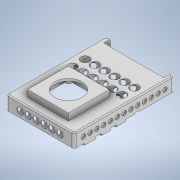
# Autodesk Inventor part: Pi 4 Case  - Upper Panel
Saved by Autodesk Inventor 2020 (Build 240168000, 168)
## iProperties
Created: 2021-01-01
Part Number: Pi 4 Case  - Upper Panel
Material: Generic
Document SubType Name: Modeling
Designer: frost
Density: 1 g/cm^3
Appearance: Default
Author: frost
Autodesk Inventor part; units mm, degrees
ref_plane "YZ Plane" through (0, 0, 0) normal (1, 0, 0) x (0, 1, 0)
ref_plane "XZ Plane" through (0, 0, 0) normal (0, 1, 0) x (-1, 0, 0)
sketch "Sketch1" plane through (0, 0, 0) normal (0, 1, 0) x (-1, 0, 0)
  line L0 (28, 44) -> (-28, 44)
  line L1 (-30, 42) -> (-30, -42)
  line L2 (-28, -44) -> (28, -44)
  line L3 (30, -42) -> (30, 42)
  line L4 (30, 44) -> (-30, -44) construction
  line L5 (-30, 44) -> (30, -44) construction
  line L6 (25, 42.5) -> (-25, 42.5)
  line L7 (-28, 39.5) -> (-28, -39.5)
  line L8 (-25, -42.5) -> (25, -42.5)
  line L9 (28, -39.5) -> (28, 39.5)
  line L10 (28, 42.5) -> (-28, -42.5) construction
  line L11 (-28, 42.5) -> (28, -42.5) construction
  arc A0 (25, -42.5) -> (28, -39.5) centre (25, -39.5) ccw
  arc A1 (-28, -39.5) -> (-25, -42.5) centre (-25, -39.5) ccw
  arc A2 (-25, 42.5) -> (-28, 39.5) centre (-25, 39.5) ccw
  arc A3 (28, 39.5) -> (25, 42.5) centre (25, 39.5) ccw
  arc A4 (-30, -42) -> (-28, -44) centre (-28, -42) ccw
  arc A5 (-28, 44) -> (-30, 42) centre (-28, 42) ccw
  arc A6 (28, -44) -> (30, -42) centre (28, -42) ccw
  arc A7 (30, 42) -> (28, 44) centre (28, 42) ccw
  point P0 (0, 0)
  dimension "d2" = 60
  dimension "d3" = 88
  dimension "d4" = 56
  dimension "d5" = 85
  dimension "d6" = 3
  dimension "d7" = 2
  constraints: 24 end point, 16 point on circle, 16 point on line, 16 tangent, 8 centre point, 6 equal radius, 4 midpoint, 4 parallel, 2 horizontal, 2 perpendicular
  measures "d2" distance of L4.end L5.end
  measures "d3" distance of L5.start L4.end
  measures "d4" distance of L11.end L10.end
  measures "d5" distance of L10.end L11.start
  measures "d6" radius of A0
  measures "d7" radius of A4
extrude "Extrusion1" add sketch "Sketch1" along normal blind 4 contours A7 L3 A6 L2 A4 L1 A5 L0 | A3 L9 A0 L8 A1 L7 A2 L6
extrude "Extrusion2" add sketch "Sketch1" against normal blind 8
sketch "Sketch2" plane through (28, 4, -44) normal (0, 0, -1) x (-1, 0, 0)
  line L0 (53, -12) -> (3, -12) projected
  line L1 (2, -1) -> (54, -1)
  line L2 (54, -1) -> (54, -12)
  line L3 (54, -12) -> (2, -12)
  line L4 (2, -12) -> (2, -1)
  line L5 (-2, -12) -> (-2, 0) projected
  line L6 (58, -12) -> (58, 0) projected
  point P0 (28, -4)
  point P1 (3, -12)
  dimension "d12" = 4
  dimension "d13" = 4
  dimension "d14" = 11
  constraints: 8 end point, 2 parallel, 1 horizontal, 1 perpendicular, 1 point on line
  measures "d12" distance between parallel lines of L5 L4
  measures "d13" distance between parallel lines of L6 L2
  measures "d14" distance of L1.end L2.end
extrude "Extrusion3" cut sketch "Sketch2" against normal blind 19
sketch "Sketch3" plane through (28, 4, -44) normal (0, 0, -1) x (-1, 0, 0)
  line L0 (2, -1) -> (54, -1) projected
  line L1 (54, -1) -> (38, -1)
  line L2 (38, -1) -> (38, -3.5)
  line L3 (38, -3.5) -> (54, -3.5)
  line L4 (54, -3.5) -> (54, -1)
  line L5 (0, 0) -> (56, 0) projected
  line L6 (2, -1) -> (54, -1)
  line L7 (54, -1) -> (54, 0)
  line L8 (54, 0) -> (2, 0)
  line L9 (2, 0) -> (2, -1)
  point P0 (28, -4)
  point P1 (38, -1)
  dimension "d67" = 6
  dimension "d17" = 16
  dimension "d18" = 2.5
  constraints: 16 end point, 4 parallel, 2 horizontal, 2 perpendicular, 1 point on line
  measures "d17" distance of L3.end L2.end
  measures "d18" distance of L2.end L1.end
extrude "Extrusion4" add sketch "Sketch3" against normal blind 21 contours L0 L4 L3 L2
extrude "Extrusion5" cut sketch "Sketch3" against normal blind 5
sketch "Sketch4" plane through (30, 4, 42) normal (1, 0, 0) x (0, 0, -1)
  line L0 (86, -12) -> (86, 0) projected
  line L1 (84, -12) -> (0, -12) projected
  circle A0 centre (53.5, -14.5) radius 3.5
  point P0 (42, -4)
  point P1 (51.05051, -12)
  point P2 (55.94949, -12)
  dimension "d27" = 2.5
  dimension "d28" = 32.5
  dimension "d29" = 7
  constraints: 1 centre point
  measures "d27" distance from line of L1 A0.centre
  measures "d28" distance from line of L0 A0.centre
  measures "d29" diameter of A0
extrude "Extrusion6" cut sketch "Sketch4" against normal blind 10 contours L1 A0 picked at (52.886513, -11.84099)
sketch "Sketch5" plane through (30, 4, 42) normal (1, 0, 0) x (0, 0, -1)
  line L0 (-4.909383, -13.7) -> (89.753099, -13.7)
  line L1 (84, -12) -> (55.94949, -12)
  point P0 (42, -4)
  dimension "d32" = 1.7
  constraints: 2 end point, 1 horizontal
  measures "d32" distance between parallel lines of L1 L0
sketch "Sketch6" plane through (30, 4, 42) normal (1, 0, 0) x (0, 0, -1)
  line L0 (43, -10.06382) -> (43, -13.7)
  arc A0 (55.94949, -12) -> (51.05051, -12) centre (53.5, -14.5) ccw
  line L1 (35, -10.06382) -> (35, -13.7)
  line L2 (30, -13.7) -> (30, -10.06382)
  line L3 (22, -10.06382) -> (22, -13.7)
  line L4 (17, -10.06382) -> (17, -13.7)
  line L5 (7, -10.06382) -> (7, -13.7)
  line L6 (6.470177, -10.06382) -> (43, -10.06382)
  line L7 (-3.727507, -13.7) -> (104.881709, -13.7)
  line L8 (84, -12) -> (55.94949, -12)
  point P0 (42, -4)
  dimension "d33" = 10.5
  dimension "d34" = 8
  dimension "d35" = 5
  dimension "d36" = 8
  dimension "d37" = 5
  dimension "d38" = 10
  dimension "d39" = 1.7
  constraints: 16 end point, 11 point on line, 6 vertical, 2 horizontal
  measures "d33" distance from line of L0 A0.centre
  measures "d34" distance between parallel lines of L0 L1
  measures "d35" distance between parallel lines of L1 L2
  measures "d36" distance between parallel lines of L3 L2
  measures "d37" distance between parallel lines of L4 L3
  measures "d38" distance between parallel lines of L4 L5
  measures "d39" distance between parallel lines of L8 L7
extrude "Extrusion7" add sketch "Sketch6" against normal blind 2 contours L0 L7 L1 L6 | L2 L7 L3 L6 | L4 L7 L5 L6
fillet "Fillet1" radius 1 11 edges at (29.4142, 4, -43.4142) (27, 4, -44) (29.4142, 4, 43.4142) (0, 4, 44) (-29.4142, 4, 43.4142) (-30, 4, 0) (-29.4142, 4, -43.4142) (-27, 4, -44) (30, 4, 0) (0, 4, -39) (26, 4, -41.5)
sketch "Sketch8" plane through (0, 0, 0) normal (0, -1, 0) x (1, 0, 0)
  line L0 (28, 44) -> (-28, 44)
  line L1 (0, 44) -> (0, 19)
  line L2 (0, 19) -> (12.020815, 31.020815)
  line L3 (0, 19) -> (16.563989, 19)
  line L4 (0, 19) -> (-12.020815, 31.020815)
  line L5 (0, 19) -> (12.020815, 6.979185)
  line L6 (0, 19) -> (-12.020815, 6.979185)
  circle A0 centre (12.020815, 31.020815) radius 1.25
  circle A1 centre (-12.020815, 31.020815) radius 1.25
  circle A2 centre (12.020815, 6.979185) radius 1.25
  circle A3 centre (-12.020815, 6.979185) radius 1.25
  line L7 (17, 36) -> (-17, 36)
  line L8 (-17, 36) -> (-17, 2)
  line L9 (-17, 2) -> (17, 2)
  line L10 (17, 2) -> (17, 36)
  line L11 (17, 36) -> (-17, 2) construction
  line L12 (-17, 36) -> (17, 2) construction
  line L13 (18, 37) -> (-18, 37)
  line L14 (-18, 37) -> (-18, 1)
  line L15 (-18, 1) -> (18, 1)
  line L16 (18, 1) -> (18, 37)
  line L17 (18, 37) -> (-18, 1) construction
  line L18 (-18, 37) -> (18, 1) construction
  circle A4 centre (-12.020815, 6.979185) radius 2.5
  circle A5 centre (-12.020815, 31.020815) radius 2.5
  circle A6 centre (12.020815, 31.020815) radius 2.5
  circle A7 centre (12.020815, 6.979185) radius 2.5
  point P0 (0, 0)
  dimension "d43" = 25
  dimension "d44" = 17
  dimension "d45" = 45
  dimension "d46" = 2.5
  dimension "d47" = 2.5
  dimension "d48" = 34
  dimension "d49" = 34
  dimension "d50" = 36
  dimension "d51" = 36
  dimension "d56" = 5
  dimension "d57" = 5
  dimension "d58" = 5
  dimension "d59" = 5
  constraints: 36 end point, 8 centre point, 5 coincident, 5 midpoint, 5 symmetric about line, 4 parallel, 3 horizontal, 2 perpendicular, 1 point on line, 1 vertical, 2 other
  measures "d43" distance of L1.start L1.end
  measures "d44" distance of L1.end L2.end
  measures "d45" angle of L1 L2
  measures "d46" diameter of A0
  measures "d47" diameter of A1
  measures "d48" distance of L9.end L8.end
  measures "d49" distance of L8.end L7.end
  measures "d50" distance of L15.end L14.end
  measures "d51" distance of L15.end L13.start
  measures "d56" diameter of A4
  measures "d57" diameter of A5
  measures "d58" diameter of A6
  measures "d59" diameter of A7
extrude "Extrusion8" add sketch "Sketch8" against normal blind 10 contours A0 | A1 | A2 | A3 | L10 L9 L8 L7 | L16 L15 L14 L13 | A4 | A5 | A6 | A7
extrude "Extrusion9" cut sketch "Sketch8" against normal blind 8 contours A0 | A1 | A2 | A3 | L10 L9 L8 L7 | A4 | A5 | A6 | A7
extrude "Extrusion10" add sketch "Sketch8" against normal blind 8 contours A4 | A5 | A6 | A7
extrude "Extrusion11" cut sketch "Sketch8" against normal blind 4 contours A4 | A5 | A6 | A7
sketch "Sketch9" plane through (0, 10, 0) normal (0, 1, 0) x (1, 0, 0)
  circle A0 centre (12.020815, -31.020815) radius 1.25
  circle A1 centre (-12.020815, -6.979185) radius 1.25
  line L0 (12.020815, -31.020815) -> (-12.020815, -6.979185)
  circle A2 centre (0, -19) radius 12
  point P0 (0, 0)
  dimension "d64" = 24
  constraints: 2 end point, 1 centre point, 1 midpoint
  measures "d64" diameter of A2
extrude "Extrusion12" cut sketch "Sketch9" against normal blind 4 contours A2 L0 | L0 A2
sketch "Sketch10" plane through (-30, -8, -42) normal (-1, 0, 0) x (0, 0, 1)
  line L0 (84, 11) -> (0, 11)
  line L1 (0, 11) -> (0, 0)
  line L2 (2.5, 0) -> (-0.328427, 0)
  line L3 (0, 0) -> (0, 11)
  line L4 (0, 5.5) -> (132, 5.5)
  circle A0 centre (6, 5.5) radius 2
  circle A1 centre (12, 5.5) radius 2
  circle A2 centre (18, 5.5) radius 2
  circle A3 centre (24, 5.5) radius 2
  circle A4 centre (30, 5.5) radius 2
  circle A5 centre (36, 5.5) radius 2
  circle A6 centre (42, 5.5) radius 2
  circle A7 centre (48, 5.5) radius 2
  circle A8 centre (54, 5.5) radius 2
  circle A9 centre (60, 5.5) radius 2
  circle A10 centre (66, 5.5) radius 2
  circle A11 centre (72, 5.5) radius 2
  circle A12 centre (78, 5.5) radius 2
  line L5 (84, 0) -> (84, 11)
  circle A13 centre (9, 5.5) radius 2
  circle A14 centre (15, 5.5) radius 2
  circle A15 centre (21, 5.5) radius 2
  circle A16 centre (27, 5.5) radius 2
  circle A17 centre (33, 5.5) radius 2
  circle A18 centre (39, 5.5) radius 2
  circle A19 centre (45, 5.5) radius 2
  circle A20 centre (51, 5.5) radius 2
  circle A21 centre (57, 5.5) radius 2
  circle A22 centre (63, 5.5) radius 2
  circle A23 centre (69, 5.5) radius 2
  circle A24 centre (75, 5.5) radius 2
  circle A25 centre (81, 5.5) radius 2
  circle A26 centre (3, 5.5) radius 2
  point P0 (42, 8)
  dimension "d67" = 6
  dimension "d68" = 6
  dimension "d69" = 6
  dimension "d70" = 6
  dimension "d71" = 6
  dimension "d72" = 6
  dimension "d73" = 6
  dimension "d74" = 6
  dimension "d75" = 6
  dimension "d76" = 6
  dimension "d77" = 6
  dimension "d78" = 6
  dimension "d79" = 6
  dimension "d80" = 4
  dimension "d81" = 3
  dimension "d82" = 3
  dimension "d83" = 3
  dimension "d84" = 3
  dimension "d85" = 3
  dimension "d86" = 3
  dimension "d87" = 3
  dimension "d88" = 3
  dimension "d89" = 3
  dimension "d90" = 3
  dimension "d91" = 3
  dimension "d92" = 3
  dimension "d93" = 3
  dimension "d94" = 3
  constraints: 27 centre point, 26 equal radius, 2 end point, 1 midpoint, 1 point on line, 1 vertical, 30 other
  measures "d67" distance from line of L1 A0.centre
  measures "d68" distance of A0.centre A1.centre
  measures "d69" distance from line of L5 A12.centre
  measures "d70" distance of A12.centre A11.centre
  measures "d71" distance of A11.centre A10.centre
  measures "d72" distance of A10.centre A9.centre
  measures "d73" distance of A9.centre A8.centre
  measures "d74" distance of A8.centre A7.centre
  measures "d75" distance of A7.centre A6.centre
  measures "d76" distance of A6.centre A5.centre
  measures "d77" distance of A5.centre A4.centre
  measures "d78" distance of A4.centre A3.centre
  measures "d79" distance of A3.centre A2.centre
  measures "d80" diameter of A0
  measures "d81" distance of A0.centre A26.centre
  measures "d82" distance of A1.centre A13.centre
  measures "d83" distance of A2.centre A14.centre
  measures "d84" distance of A3.centre A15.centre
  measures "d85" distance of A4.centre A16.centre
  measures "d86" distance of A5.centre A17.centre
  measures "d87" distance of A6.centre A18.centre
  measures "d88" distance of A7.centre A19.centre
  measures "d89" distance of A8.centre A20.centre
  measures "d90" distance of A9.centre A21.centre
  measures "d91" distance of A10.centre A22.centre
  measures "d92" distance of A11.centre A23.centre
  measures "d93" distance of A12.centre A24.centre
  measures "d94" distance of A12.centre A25.centre
extrude "Extrusion13" cut sketch "Sketch10" against normal blind 3 contours A25 A12 L4 | L4 A12 A25 | A26 A0 L4 | L4 A0 A26 | A12 A25 L4 | L4 A25 A12 | A0 A26 L4 | L4 A26 A0 | A24 L4 A12 | A12 L4 A11 A24 | A24 A11 L4 A12 | A12 L4 A24 | A13 A1 L4 A0 | A0 L4 A13 | A13 L4 A0 | A0 L4 A1 A13 | A11 L4 A24 | A24 L4 A11 | A13 L4 A1 | A1 L4 A13 | A23 L4 A11 | A11 L4 A10 A23 | A23 A10 L4 A11 | A11 L4 A23 | A14 A2 L4 A1 | A1 L4 A14 | A14 L4 A1 | A1 L4 A2 A14 | A10 L4 A23 | A23 L4 A10 | A14 L4 A2 | A2 L4 A14 | A22 L4 A10 | A10 L4 A9 A22 | A22 A9 L4 A10 | A10 L4 A22 | A15 A3 L4 A2 | A2 L4 A15 | A15 L4 A2 | A2 L4 A3 A15 | A9 L4 A22 | A22 L4 A9 | A15 L4 A3 | A3 L4 A15 | A21 L4 A9 | A9 L4 A8 A21 | A21 A8 L4 A9 | A9 L4 A21 | A16 A4 L4 A3 | A3 L4 A16 | A16 L4 A3 | A3 L4 A4 A16 | A8 L4 A21 | A21 L4 A8 | A16 L4 A4 | A4 L4 A16 | A20 L4 A8 | A8 L4 A7 A20 | A20 A7 L4 A8 | A8 L4 A20 | A17 A5 L4 A4 | A4 L4 A17 | A17 L4 A4 | A4 L4 A5 A17 | A7 L4 A20 | A20 L4 A7 | A17 L4 A5 | A5 L4 A17 | A19 L4 A7 | A7 L4 A6 A19 | A19 A6 L4 A7 | A7 L4 A19 | A18 A6 L4 A5 | A5 L4 A18 | A18 L4 A5 | A5 L4 A6 A18 | A6 L4 A19 | A19 L4 A6 | A18 L4 A6 | A6 L4 A18
extrude "Extrusion14" add sketch "Sketch10" against normal blind 1 contours A25 A12 L4 | L4 A12 A25 | A26 A0 L4 | L4 A0 A26 | A12 A25 L4 | L4 A25 A12 | A0 A26 L4 | L4 A26 A0 | A24 L4 A12 | A12 L4 A11 A24 | A24 A11 L4 A12 | A12 L4 A24 | A13 A1 L4 A0 | A0 L4 A13 | A13 L4 A0 | A0 L4 A1 A13 | A11 L4 A24 | A24 L4 A11 | A13 L4 A1 | A1 L4 A13 | A23 L4 A11 | A11 L4 A10 A23 | A23 A10 L4 A11 | A11 L4 A23 | A14 A2 L4 A1 | A1 L4 A14 | A14 L4 A1 | A1 L4 A2 A14 | A10 L4 A23 | A23 L4 A10 | A14 L4 A2 | A2 L4 A14 | A22 L4 A10 | A10 L4 A9 A22 | A22 A9 L4 A10 | A10 L4 A22 | A15 A3 L4 A2 | A2 L4 A15 | A15 L4 A2 | A2 L4 A3 A15 | A9 L4 A22 | A22 L4 A9 | A15 L4 A3 | A3 L4 A15 | A21 L4 A9 | A9 L4 A8 A21 | A21 A8 L4 A9 | A9 L4 A21 | A16 A4 L4 A3 | A3 L4 A16 | A16 L4 A3 | A3 L4 A4 A16 | A8 L4 A21 | A21 L4 A8 | A16 L4 A4 | A4 L4 A16 | A20 L4 A8 | A8 L4 A7 A20 | A20 A7 L4 A8 | A8 L4 A20 | A17 A5 L4 A4 | A4 L4 A17 | A17 L4 A4 | A4 L4 A5 A17 | A7 L4 A20 | A20 L4 A7 | A17 L4 A5 | A5 L4 A17 | A19 L4 A7 | A7 L4 A6 A19 | A19 A6 L4 A7 | A7 L4 A19 | A18 A6 L4 A5 | A5 L4 A18 | A18 L4 A5 | A5 L4 A6 A18 | A6 L4 A19 | A19 L4 A6 | A18 L4 A6 | A6 L4 A18
extrude "Extrusion15" cut sketch "Sketch10" against normal blind 1 contours A12 A25 L4 | L4 A25 A12 | A25 L4 A24 A12 | A12 A24 L4 A25 | A0 A26 L4 | L4 A26 A0 | A0 A13 L4 A26 | A26 L4 A13 A0 | A24 L4 A12 | A12 L4 A24 | A0 L4 A13 | A13 L4 A0 | A24 L4 A23 A11 | A11 L4 A24 | A24 L4 A11 | A11 A23 L4 A24 | A13 L4 A1 | A1 A14 L4 A13 | A13 L4 A14 A1 | A1 L4 A13 | A23 L4 A11 | A11 L4 A23 | A1 L4 A14 | A14 L4 A1 | A23 L4 A22 A10 | A10 L4 A23 | A23 L4 A10 | A10 A22 L4 A23 | A14 L4 A2 | A2 A15 L4 A14 | A14 L4 A15 A2 | A2 L4 A14 | A22 L4 A10 | A10 L4 A22 | A2 L4 A15 | A15 L4 A2 | A22 L4 A21 A9 | A9 L4 A22 | A22 L4 A9 | A9 A21 L4 A22 | A15 L4 A3 | A3 A16 L4 A15 | A15 L4 A16 A3 | A3 L4 A15 | A21 L4 A9 | A9 L4 A21 | A3 L4 A16 | A16 L4 A3 | A21 L4 A20 A8 | A8 L4 A21 | A21 L4 A8 | A8 A20 L4 A21 | A16 L4 A4 | A4 A17 L4 A16 | A16 L4 A17 A4 | A4 L4 A16 | A20 L4 A8 | A8 L4 A20 | A4 L4 A17 | A17 L4 A4 | A20 L4 A19 A7 | A7 L4 A20 | A20 L4 A7 | A7 A19 L4 A20 | A17 L4 A5 | A5 A18 L4 A17 | A17 L4 A18 A5 | A5 L4 A17 | A19 L4 A7 | A7 L4 A19 | A5 L4 A18 | A18 L4 A5 | A19 L4 A18 A6 | A6 L4 A19 | A19 L4 A6 | A6 A18 L4 A19 | A18 L4 A6 | A6 L4 A18 picked at (79.352586, 5.340941) picked at (79.352586, 5.659059) picked at (4.352586, 5.659059) picked at (4.352586, 5.340941)
ref_plane "Work Plane1" through (0, -8, -42) normal (-1, 0, 0) x (0, 0, 1)
mirror "Mirror1" about plane through (0, -8, -42) normal (-1, 0, 0) of "Extrusion15", "Extrusion14", "Extrusion13"
sketch "Sketch11" plane through (-28, -8, 44) normal (0, 0, 1) x (1, 0, 0)
  line L0 (0, 11) -> (-2, 11)
  line L1 (0, 0) -> (0, 11)
  line L2 (0, 11) -> (0, 0)
  line L3 (0, 7.5) -> (0, 3.5)
  line L4 (0, 5.5) -> (67.775068, 5.5)
  circle A0 centre (7, 5.5) radius 3
  circle A1 centre (14, 5.5) radius 3
  circle A2 centre (21, 5.5) radius 3
  circle A3 centre (28, 5.5) radius 3
  circle A4 centre (35, 5.5) radius 3
  circle A5 centre (42, 5.5) radius 3
  circle A6 centre (49, 5.5) radius 3
  line L5 (56, 11) -> (56, 0)
  circle A7 centre (45.5, 5.5) radius 3
  circle A8 centre (38.5, 5.5) radius 3
  circle A9 centre (31.5, 5.5) radius 3
  circle A10 centre (24.5, 5.5) radius 3
  circle A11 centre (10.5, 5.5) radius 3
  circle A12 centre (17.5, 5.5) radius 3
  point P0 (28, 8)
  dimension "d101" = 7
  dimension "d102" = 7
  dimension "d103" = 7
  dimension "d104" = 7
  dimension "d105" = 7
  dimension "d106" = 7
  dimension "d107" = 7
  dimension "d108" = 6
  dimension "d109" = 3.5
  dimension "d110" = 3.5
  dimension "d111" = 3.5
  dimension "d112" = 3.5
  dimension "d113" = 3.5
  dimension "d114" = 3.5
  constraints: 13 centre point, 12 equal radius, 2 end point, 1 collinear, 1 midpoint, 16 other
  measures "d101" distance from line of L1 A0.centre
  measures "d102" distance of A1.centre A0.centre
  measures "d103" distance of A1.centre A2.centre
  measures "d104" distance from line of L5 A6.centre
  measures "d105" distance of A6.centre A5.centre
  measures "d106" distance of A5.centre A4.centre
  measures "d107" distance of A4.centre A3.centre
  measures "d108" diameter of A0
  measures "d109" distance of A1.centre A11.centre
  measures "d110" distance of A2.centre A12.centre
  measures "d111" distance of A3.centre A10.centre
  measures "d112" distance of A4.centre A9.centre
  measures "d113" distance of A5.centre A8.centre
  measures "d114" distance of A6.centre A7.centre
extrude "Extrusion16" cut sketch "Sketch11" against normal blind 1.5 contours A7 A6 L4 | A7 A6 L4 | L4 A6 A7 | L4 A6 A7 | A5 A7 L4 | L4 A7 A5 | A7 L4 A8 A5 | A5 A8 L4 A7 | A8 L4 A5 | A5 L4 A8 | A8 L4 A9 A4 | A4 L4 A8 | A8 L4 A4 | A4 A9 L4 A8 | A9 L4 A4 | A4 L4 A9 | A9 L4 A10 A3 | A3 L4 A9 | A9 L4 A3 | A3 A10 L4 A9 | A10 L4 A3 | A3 L4 A10 | A10 L4 A12 A2 | A2 L4 A10 | A10 L4 A2 | A2 A12 L4 A10 | A12 L4 A2 | A2 L4 A12 | A12 L4 A11 A1 | A1 L4 A12 | A12 L4 A1 | A1 A11 L4 A12 | A11 L4 A1 | A1 L4 A11 | A11 L4 A0 | A0 L4 A11 | A11 L4 A0 | A0 L4 A11
extrude "Extrusion17" add sketch "Sketch11" against normal blind 0.75 contours A7 A6 L4 | A7 A6 L4 | L4 A6 A7 | L4 A6 A7 | A5 A7 L4 | L4 A7 A5 | A7 L4 A8 A5 | A5 A8 L4 A7 | A8 L4 A5 | A5 L4 A8 | A8 L4 A9 A4 | A4 L4 A8 | A8 L4 A4 | A4 A9 L4 A8 | A9 L4 A4 | A4 L4 A9 | A9 L4 A10 A3 | A3 L4 A9 | A9 L4 A3 | A3 A10 L4 A9 | A10 L4 A3 | A3 L4 A10 | A10 L4 A12 A2 | A2 L4 A10 | A10 L4 A2 | A2 A12 L4 A10 | A12 L4 A2 | A2 L4 A12 | A12 L4 A11 A1 | A1 L4 A12 | A12 L4 A1 | A1 A11 L4 A12 | A11 L4 A1 | A1 L4 A11 | A11 L4 A0 | A0 L4 A11 | A11 L4 A0 | A0 L4 A11
extrude "Extrusion18" cut sketch "Sketch11" against normal blind 0.75 contours A7 A6 L4 | L4 A6 A7 | A6 A7 A5 L4 | L4 A5 A7 A6 | A5 A7 L4 | L4 A7 A5 | A8 L4 A5 | A5 L4 A4 A8 | A8 A4 L4 A5 | A5 L4 A8 | A4 L4 A8 | A8 L4 A4 | A9 L4 A4 | A4 L4 A3 A9 | A9 A3 L4 A4 | A4 L4 A9 | A3 L4 A9 | A9 L4 A3 | A10 L4 A3 | A3 L4 A2 A10 | A10 A2 L4 A3 | A3 L4 A10 | A2 L4 A10 | A10 L4 A2 | A12 L4 A2 | A2 L4 A1 A12 | A12 A1 L4 A2 | A2 L4 A12 | A1 L4 A12 | A12 L4 A1 | A11 L4 A1 | A1 L4 A0 A11 | A11 A0 L4 A1 | A1 L4 A11 | A0 L4 A11 | A11 L4 A0 picked at (46.861285, 5.26522) picked at (46.861285, 5.73478) picked at (9.138715, 5.73478) picked at (9.138715, 5.26522)
sketch "Sketch14" plane through (0, 0, 0) normal (0, -1, 0) x (1, 0, 0)
  line L0 (0, 0) -> (-25, 0)
  line L1 (-25, 0) -> (-25, -18)
  line L2 (-25, -18) -> (0, -18)
  line L3 (0, -18) -> (0, 0)
  line L4 (0, 0) -> (25, 0)
  line L5 (25, 0) -> (25, -18)
  line L6 (25, -18) -> (0, -18)
  line L7 (34.785047, -4.5) -> (-36.800059, -4.5)
  line L8 (35.821511, -12) -> (-40.324037, -12)
  circle A0 centre (0, -4.5) radius 3.75
  line L9 (34.785047, -19.5) -> (-36.800059, -19.5)
  circle A1 centre (0, -19.5) radius 3.75
  line L10 (0, -4.5) -> (4.330127, -12)
  line L11 (4.330127, -12) -> (8.660254, -4.5)
  line L12 (8.660254, -4.5) -> (12.990381, -12)
  line L13 (12.990381, -12) -> (17.320508, -4.5)
  line L14 (17.320508, -4.5) -> (21.650635, -12)
  line L15 (21.650635, -12) -> (24.537386, -7)
  line L16 (24.537386, -7) -> (27.424138, -12)
  line L17 (27.424138, -12) -> (31.754265, -4.5)
  circle A2 centre (4.330127, -12) radius 3.75
  circle A3 centre (8.660254, -4.5) radius 3.75
  circle A4 centre (12.999808, -12) radius 3.75
  circle A5 centre (17.320508, -4.5) radius 3.75
  circle A6 centre (21.650635, -12) radius 3.75
  circle A7 centre (8.660254, -19.5) radius 3.75
  circle A8 centre (17.320508, -19.5) radius 3.75
  line L18 (8.660254, -0.75) -> (8.660254, -8.25)
  line L19 (17.320508, -0.75) -> (17.320508, -8.25)
  line L20 (4.400827, -8.250667) -> (4.400827, -15.749333)
  line L21 (13.070508, -8.250667) -> (13.070508, -15.749333)
  line L22 (21.721335, -8.250667) -> (21.721335, -15.749333)
  line L23 (17.320508, -15.75) -> (17.320508, -23.25)
  line L24 (8.660254, -15.75) -> (8.660254, -23.25)
  line L25 (0, -23.25) -> (0, -15.75)
  circle A9 centre (4.410254, -6.75) radius 3.75
  circle A10 centre (13.070508, -6.5) radius 3.75
  circle A11 centre (21.730762, -6.5) radius 3.75
  line L26 (4.410254, -3) -> (4.410254, -21.453739)
  line L27 (13.070508, -21.203739) -> (13.070508, -2.75)
  line L28 (21.730762, -2.75) -> (21.730762, -21.203739)
  circle A12 centre (4.410254, -17.25) radius 3.75
  circle A13 centre (13.070508, -17.5) radius 3.75
  circle A14 centre (21.730762, -17.5) radius 3.75
  point P0 (0, -0.75)
  point P1 (0, -8.25)
  point P2 (4.400827, -12)
  point P3 (4.400827, -11.877543)
  point P4 (13.070508, -11.861216)
  point P5 (13.070508, -12)
  point P6 (21.721335, -11.877543)
  point P7 (21.721335, -12)
  dimension "d152" = 25
  dimension "d153" = 18
  dimension "d154" = 7.5
  dimension "d155" = 4.5
  dimension "d156" = 7.5
  dimension "d158" = 60
  dimension "d159" = 60
  dimension "d205" = 0
  constraints: 58 end point, 16 point on circle, 15 point on line, 12 centre point, 12 parallel, 9 symmetric about line, 6 equal radius, 4 coincident, 3 horizontal, 3 perpendicular, 3 vertical alignment, 1 vertical, 14 other
  measures "d152" distance of L2.end L1.end
  measures "d153" distance of L1.end L0.end
  measures "d154" diameter of A0
  measures "d155" distance between parallel lines of L0 L7
  measures "d156" distance between parallel lines of L7 L8
  measures "d158" angle of L7 L10
  measures "d159" angle of L11 L10
  measures "d205" distance from line of L8 A4.centre
revolve "Revolution18" cut sketch "Sketch14" angle 360 about axis through (0, 0, -18) along (0, 0, 1) contours L3 L7 A0 | L3 A0 L7 | A1 L3 L2 | L2 L25 L9 A1 | L9 L25 A1
revolve "Revolution19" cut sketch "Sketch14" angle 360 about axis through (8.660254, 0, -15.75) along (0, 0, -1) contours A9 L7 A3 | A3 L18 L7 A9 | L7 A9 L11 A3 | L7 L11 A9 | L11 A9 A3 | L18 A3 A9 L11 | A7 A12 L6 | L6 A12 L9 A7 | A12 L9 L24 A7 | A7 L9 A12 | A12 A7 L24 L6 | L6 L24 L9 A12
revolve "Revolution20" cut sketch "Sketch14" angle 360 about axis through (17.320508, 0, -15.75) along (0, 0, -1) contours L19 L7 A10 A5 | L13 A10 L7 | L19 A5 A10 L13 | A10 L7 A5 | A10 L13 A5 L7 | A10 A5 L13 | A8 A13 L9 L23 | L23 L6 A13 A8 | L23 L9 A13 L6 | A8 L9 A13 | A13 L6 A8 | L6 A13 L9 A8
revolve "Revolution21" cut sketch "Sketch14" angle 360 about axis through (4.410254, 0, -3) along (0, 0, -1) contours A2 A9 L10 L8 | L8 L20 A12 A2 | A2 L10 A9 | A2 L20 A9 L10 | L10 A9 L20 L11 | A12 L20 A2
revolve "Revolution22" cut sketch "Sketch14" angle 360 about axis through (13.070508, 0, -21.203739) along (0, 0, 1) picked at (11.333591, -12.931983) picked at (12.834327, -14.43896) contours A4 A10 L12 L8 | L8 L21 A13 A4 | L21 A10 L12 A4 | L12 A10 A4 | L12 A10 L21 L13 | A13 L21 A4
revolve "Revolution23" cut sketch "Sketch14" angle 360 about axis through (21.730762, 0, -2.75) along (0, 0, -1) contours L22 A11 L14 A6 | L14 A11 A6 | L22 L15 L14 A11 | L22 A14 A6 L8 | L14 L8 A6 A11 | L22 A6 A14
sketch "Sketch17" plane through (0, 4, 0) normal (0, 1, 0) x (1, 0, 0)
  point P0 (0, 0)
sketch "Sketch18" plane through (0, 4, 0) normal (0, 1, 0) x (1, 0, 0)
  point P0 (0, 0)
sketch "Sketch19" plane through (0, 4, 0) normal (0, 1, 0) x (1, 0, 0)
  circle A0 centre (4.410254, 6.75) radius 3.75
  circle A1 centre (13.070508, 6.5) radius 3.75
  circle A2 centre (21.730762, 6.5) radius 3.75
  circle A3 centre (21.730762, 17.5) radius 3.75
  circle A4 centre (13.070508, 17.5) radius 3.75
  circle A5 centre (4.410254, 17.25) radius 3.75
  line L0 (4.410254, 3) -> (4.410254, 21.453739)
  line L1 (13.070508, 2.75) -> (13.070508, 21.25)
  line L2 (21.730762, 21.25) -> (21.730762, 3)
  line L3 (21.730762, 3) -> (21.730762, 2.75)
  point P0 (0, 0)
  point P1 (21.730762, 13.75)
  point P2 (21.730762, 10.25)
  point P3 (13.070508, 13.75)
  point P4 (13.070508, 10.25)
  point P5 (4.410254, 21)
  point P6 (4.410254, 13.5)
  point P7 (4.410254, 10.5)
  constraints: 6 end point, 1 parallel, 1 point on line, 1 vertical, 9 other
revolve "Revolution24" cut sketch "Sketch19" angle 360 about axis through (21.730762, 4, -21.25) along (0, 0, 1) picked at (22.008913, 7.801993) picked at (22.986203, 18.248022) contours L3 L2 A2 | A3 L2
revolve "Revolution25" cut sketch "Sketch19" angle 360 about axis through (13.070508, 4, -2.75) along (0, 0, -1) picked at (13.84987, 7.477289) picked at (14.325949, 18.248022) contours L1 A1 | A4 L1
revolve "Revolution26" cut sketch "Sketch19" angle 360 about axis through (4.410254, 4, -3) along (0, 0, -1) picked at (5.189616, 7.727289) picked at (6.713623, 17.528151) contours L0 A0 | A5 L0
mirror "Mirror4" about plane through (0, -8, -42) normal (-1, 0, 0) of "Revolution24", "Revolution25", "Revolution26", "Revolution18", "Revolution19", "Revolution20", "Revolution22", "Revolution21", "Revolution23"
body "Solid1"
